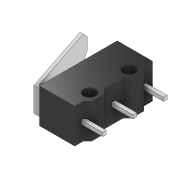
# Autodesk Inventor part: Microswitch
Saved by Autodesk Inventor 2020 (Build 240168000, 168)
## iProperties
Created: 2020-10-17
Part Number: Microswitch
Material: Generic
Document SubType Name: Modeling
Designer: ferrerx
Density: 1 g/cm^3
Appearance: Default
Mass: 0.439958 g
Surface Area: 5.81076 cm^2
Volume: 0.439958 cm^3
Author: ferrerx
Autodesk Inventor part; units mm, degrees
ref_plane "YZ Plane" through (0, 0, 0) normal (1, 0, 0) x (0, 1, 0)
ref_plane "XZ Plane" through (0, 0, 0) normal (0, 1, 0) x (-1, 0, 0)
sketch "Sketch1" plane through (0, 0, 0) normal (0, 1, 0) x (-1, 0, 0)
  line L0 (0, 0) -> (5.8, 0)
  line L1 (5.8, 0) -> (5.8, -12.8)
  line L2 (5.8, -12.8) -> (0, -12.8)
  line L3 (0, -12.8) -> (0, 0)
  dimension "d0" = 5.8
  dimension "d1" = 12.8
  constraints: 8 end point, 2 parallel, 1 horizontal, 1 perpendicular
  measures "d0" distance of L1.end L2.end
  measures "d1" distance of L0.end L1.end
extrude "Extrusion1" add sketch "Sketch1" along normal blind 5.7
sketch "Sketch2" plane through (0, 5.7, 0) normal (0, 1, 0) x (1, 0, 0)
  circle A0 centre (-1.4, 3.15) radius 1
  line L0 (-5.8, 12.8) -> (-5.8, 0) projected
  line L1 (-5.8, 6.4) -> (0, 6.4) construction
  line L2 (0, 0) -> (0, 12.8) projected
  circle A1 centre (-1.4, 9.65) radius 1
  dimension "d4" = 2
  dimension "d5" = 3.25
  dimension "d6" = 1.4
  constraints: 2 centre point, 2 end point, 2 midpoint, 1 symmetric about line, 1 other
  measures "d4" diameter of A0
  measures "d5" distance from line of L1 A0.centre
  measures "d6" distance from line of L2 A0.centre
extrude "Extrusion2" [suppressed]
sketch "Sketch3" plane through (0, 5.7, 0) normal (0, 1, 0) x (1, 0, 0)
  line L0 (0, 0) -> (0, 12.8) projected
  line L1 (0, 2.15) -> (0.7, 2.15)
  line L2 (0.7, 2.15) -> (0.7, 4.15)
  line L3 (0.7, 4.15) -> (0, 4.15)
  line L4 (0, 4.15) -> (0, 2.15)
  line L5 (0, 6.4) -> (-5.8, 6.4) construction
  line L6 (-5.8, 12.8) -> (-5.8, 0) projected
  circle A0 centre (-1.4, 3.15) radius 1 projected
  line L7 (-1.4, 3.15) -> (-5.8, 3.15) construction
  line L8 (0.7, 3.15) -> (0, 3.15) construction
  line L9 (0, 10.65) -> (0.7, 10.65)
  line L10 (0.7, 10.65) -> (0.7, 8.65)
  line L11 (0.7, 8.65) -> (0, 8.65)
  line L12 (0, 8.65) -> (0, 10.65)
  line L13 (0.7, 9.65) -> (0, 9.65) construction
  point P0 (0, 8.65)
  point P1 (0, 4.15)
  dimension "d9" = 0.7
  dimension "d10" = 2
  constraints: 24 end point, 6 symmetric about line, 4 midpoint, 2 horizontal, 2 parallel, 2 point on line, 1 collinear, 1 perpendicular
  measures "d9" distance between parallel lines of L0 L2
  measures "d10" distance of L1.end L2.end
extrude "Extrusion3" add sketch "Sketch3" against normal blind 5.7 contours L0 L9 L10 L11 | L0 L3 L2 L1
chamfer "Chamfer1" distance 0.7 angle 45 4 edges at (0, 2.85, -4.15) (0, 2.85, -10.65) (0, 2.85, -8.65) (0, 2.85, -2.15)
sketch "Sketch4" plane through (0, 5.7, 0) normal (0, 1, 0) x (1, 0, 0)
  line L0 (0.7, 4.15) -> (0.7, 2.15) projected
  line L1 (0.7, 3.15) -> (-0.7, 3.15) construction
  circle A0 centre (-0.7, 3.15) radius 1
  line L2 (0, 4.85) -> (0, 7.95) projected
  line L3 (0, 6.4) -> (-5.8, 6.4) construction
  line L4 (-5.8, 12.8) -> (-5.8, 0) projected
  circle A1 centre (-0.7, 9.65) radius 1
  point P0 (0, 0)
  dimension "d16" = 2
  dimension "d17" = 1.4
  constraints: 4 end point, 3 midpoint, 2 centre point, 1 coincident, 1 horizontal, 1 symmetric about line, 1 other
  measures "d16" diameter of A0
  measures "d17" distance of L1.start L1.end
extrude "Extrusion4" cut sketch "Sketch4" against normal blind 5.7
sketch "Sketch7" plane through (0, 0, -4.85) normal (1, 0, 0) x (0, 0, -1)
  line L0 (7.95, 5.7) -> (-4.85, 5.7) projected
  line L1 (1.55, 5.7) -> (1.55, 0) construction
  line L2 (1.25, 2.55) -> (1.85, 2.55)
  line L3 (1.85, 2.55) -> (1.85, 3.15)
  line L4 (1.85, 3.15) -> (1.25, 3.15)
  line L5 (1.25, 3.15) -> (1.25, 2.55)
  line L6 (1.25, 2.55) -> (1.85, 3.15) construction
  line L7 (1.85, 2.55) -> (1.25, 3.15) construction
  point P0 (-4.85, 0)
  point P1 (1.55, 2.85)
  dimension "d24" = 0.6
  dimension "d25" = 0.6
  constraints: 14 end point, 4 midpoint, 2 parallel, 1 horizontal, 1 perpendicular, 1 vertical
  measures "d24" distance of L2.end L3.end
  measures "d25" distance of L2.start L2.end
extrude "Extrusion6" add sketch "Sketch7" along normal blind 3.5
pattern_linear "Rectangular Pattern1" count 2 spacing 5 along (0, 0, -1) count 2 spacing 5 along (0, 0, 1) of "Extrusion6"
ref_plane "Work Plane1" through (0, 2.85, 0) normal (0, 1, 0) x (1, 0, 0)
sketch "Sketch8" plane through (0, 2.85, 0) normal (0, 1, 0) x (1, 0, 0)
  line L0 (-5.8, 12.8) -> (-5.8, 0) projected
  line L1 (-5.8, 0.4613) -> (-7.1649, 0.4613)
  line L2 (-7.1649, 0.4613) -> (-11.2583, 12.8)
  line L3 (-11.2583, 12.8) -> (-10.7315, 12.8)
  line L4 (-10.7315, 12.8) -> (-6.804, 0.9613)
  line L5 (-6.804, 0.9613) -> (-5.8, 0.9613)
  line L6 (0, 12.8) -> (-5.8, 12.8) projected
  point P0 (0, 0)
  dimension "d36" = 0.5
  dimension "d37" = 0.5
  dimension "d38" = 13
  constraints: 10 end point, 3 parallel, 2 point on line, 1 collinear, 1 perpendicular
  measures "d36" distance between parallel lines of L2 L4
  measures "d37" distance between parallel lines of L1 L5
  measures "d38" distance of L1.end L2.end
extrude "Extrusion7" add sketch "Sketch8" along normal mid plane 4
chamfer "Chamfer2" distance 1 angle 45 2 edges at (-10.9949, 4.85, -12.8) (-10.9949, 0.85, -12.8)
body "Solid1"
